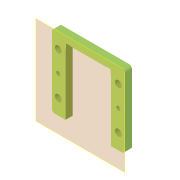
# Autodesk Inventor part: 30_Linear_Stage_NEMA11_China_lid_universal_extender_v2
Saved by Autodesk Inventor 2022 (Build 260153000, 153)
## iProperties
Created: 2022-02-11
Part Number: 30_Linear_Stage_NEMA11_China_lid_universal_extender_v2
Material: Generic
Document SubType Name: Modeling
Designer: wanghaoran
Density: 1 g/cm^3
Appearance: ipht green
Catalog Web Link: isPrinted
Vendor: openUC2
Mass: 6.04917 g
Surface Area: 45.2263 cm^2
Volume: 6.04917 cm^3
Author: wanghaoran
Autodesk Inventor part; units mm, degrees
ref_plane "YZ Plane" through (0, 0, 0) normal (1, 0, 0) x (0, 1, 0)
ref_plane "XZ Plane" through (0, 0, 0) normal (0, 1, 0) x (-1, 0, 0)
ref_plane "XY Plane" through (0, 0, 0) normal (0, 0, 1) x (1, 0, 0)
sketch "Sketch1" plane through (0, 0, 0) normal (0, 0, 1) x (1, 0, 0)
  circle A0 centre (-21, 1.215) radius 1.4 projected
  circle A1 centre (21, 1.215) radius 1.4 projected
  arc A2 (24.9, 3.115) -> (22.9, 5.115) centre (22.9, 3.115) ccw projected
  line L0 (22.9, 5.115) -> (-22.9, 5.115) projected
  arc A3 (-22.9, 5.115) -> (-24.9, 3.115) centre (-22.9, 3.115) ccw projected
  line L1 (-24.9, 3.115) -> (-24.9, -5.115) projected
  line L2 (22.8395, -5.115) -> (24.9, -5.115) projected
  line L3 (24.9, -5.115) -> (24.9, 3.115) projected
  arc A4 (22.9, -44.685) -> (24.9, -42.685) centre (22.9, -42.685) ccw projected
  line L4 (24.9, -42.685) -> (24.9, -36.885) projected
  line L5 (24.9, -36.885) -> (17.1, -36.885) projected
  line L6 (17.1, -36.885) -> (17.1, -44.685) projected
  line L7 (17.1, -44.685) -> (22.9, -44.685) projected
  circle A5 centre (21, -40.785) radius 1.4 projected
  arc A6 (-24.9, -42.685) -> (-22.9, -44.685) centre (-22.9, -42.685) ccw projected
  line L8 (-22.9, -44.685) -> (-17.1, -44.685) projected
  line L9 (-17.1, -44.685) -> (-17.1, -36.885) projected
  line L10 (-17.1, -36.885) -> (-24.9, -36.885) projected
  line L11 (-24.9, -36.885) -> (-24.9, -42.685) projected
  circle A7 centre (-21, -40.785) radius 1.4 projected
  line L12 (24.9, 5.115) -> (-24.9, 5.115)
  line L13 (-24.9, 5.115) -> (-24.9, -44.685)
  line L14 (-24.9, -44.685) -> (24.9, -44.685)
  line L15 (24.9, -44.685) -> (24.9, 5.115)
  line L16 (17.1, -2.685) -> (-17.1, -2.685)
  line L17 (-17.1, -2.685) -> (-17.1, -36.885)
  line L18 (-17.1, -36.885) -> (17.1, -36.885)
  line L19 (17.1, -36.885) -> (17.1, -2.685)
  line L20 (17.1, -36.885) -> (17.1, -44.685)
  line L21 (-17.1, -36.885) -> (-17.1, -44.685)
  circle A8 centre (0, 1.415) radius 1.4 projected
  arc A9 (-18.2605, -5.115) -> (-22.8395, -5.115) centre (-20.55, -5.335) ccw projected
  arc A10 (22.8395, -5.115) -> (18.2605, -5.115) centre (20.55, -5.335) ccw projected
  circle A11 centre (14.45, 0.765) radius 2.3 projected
  circle A12 centre (-14.45, 0.765) radius 2.3 projected
  line L22 (-24.9, -5.115) -> (-22.8395, -5.115) projected
  line L23 (-18.2605, -5.115) -> (18.2605, -5.115) projected
  circle A13 centre (20, -39.785) radius 1.4 projected
  circle A14 centre (-20, -39.785) radius 1.4 projected
  circle A15 centre (-14.45, -40.335) radius 2.3 projected
  circle A16 centre (20.55, -34.235) radius 2.3 projected
  circle A17 centre (-20.55, -34.235) radius 2.3 projected
  circle A18 centre (14.45, -40.335) radius 2.3 projected
  arc A19 (22.9, -44.685) -> (24.9, -42.685) centre (22.9, -42.685) ccw projected
  line L24 (24.9, -42.685) -> (24.9, -4.885) projected
  line L25 (24.9, -4.885) -> (22.8055, -4.885) projected
  line L26 (17.1, -4.885) -> (17.1, -36.885) projected
  line L27 (17.1, -36.885) -> (-17.1, -36.885) projected
  line L28 (-17.1, -36.885) -> (-17.1, -4.885) projected
  line L29 (-22.8055, -4.885) -> (-24.9, -4.885) projected
  line L30 (-24.9, -4.885) -> (-24.9, -42.685) projected
  arc A20 (-24.9, -42.685) -> (-22.9, -44.685) centre (-22.9, -42.685) ccw projected
  line L31 (-22.9, -44.685) -> (22.9, -44.685) projected
  arc A21 (-22.8055, -4.885) -> (-18.2945, -4.885) centre (-20.55, -5.335) ccw projected
  arc A22 (18.2945, -4.885) -> (22.8055, -4.885) centre (20.55, -5.335) ccw projected
  line L32 (18.2945, -4.885) -> (17.1, -4.885) projected
  line L33 (-17.1, -4.885) -> (-18.2945, -4.885) projected
  line L34 (17.1, -44.685) -> (15.6, -44.685)
  line L35 (15.6, -44.685) -> (15.6, -2.685)
  line L36 (15.6, -2.685) -> (17.1, -2.685)
  line L37 (17.1, -2.685) -> (17.1, -44.685)
  line L38 (-17.1, -44.685) -> (-15.6, -44.685)
  line L39 (-15.6, -44.685) -> (-15.6, -2.685)
  line L40 (-15.6, -2.685) -> (-17.1, -2.685)
  line L41 (-17.1, -2.685) -> (-17.1, -44.685)
  line L42 (-15, -27.435) -> (15, -27.435) projected
  line L43 (15, -27.435) -> (15, 0.565) projected
  line L44 (15, 0.565) -> (-15, 0.565) projected
  line L45 (-15, 0.565) -> (-15, -27.435) projected
  circle A23 centre (0, -19.785) radius 6.5 projected
  circle A24 centre (-10, -2.435) radius 2.75 projected
  circle A25 centre (10, -2.435) radius 2.75 projected
  line L46 (15.2, 0.765) -> (15.2, -27.635)
  line L47 (15.2, -27.635) -> (-15.2, -27.635)
  line L48 (-15.2, -27.635) -> (-15.2, 0.765)
  line L49 (-15.2, 0.765) -> (15.2, 0.765)
  point P0 (0, 0)
  point P1 (-20.55, -5.335)
  point P2 (20.55, -5.335)
  point P3 (-20.55, -5.335)
  point P4 (20.55, -5.335)
  point P5 (15.2, -2.685)
  point P6 (-15.2, -2.685)
  point P7 (-12.15, 0.765)
  point P8 (-12.1587, 0.565)
  point P9 (12.1587, 0.565)
  point P10 (12.15, 0.765)
  point P11 (-15.6, -36.885)
  point P12 (15.6, -36.885)
  dimension "d0" = 7.8
  dimension "d23" = 1.5
  dimension "d24" = 1.5
  dimension "d57" = 0.2
  constraints: 44 end point, 10 equal length, 7 point on line, 4 perpendicular, 3 horizontal, 6 other
  measures "d0" distance between parallel lines of L15 L19
  measures "d23" distance between parallel lines of L6 L35
  measures "d24" distance between parallel lines of L39 L28
  measures "d57" distance between parallel lines of L43 L46
extrude "Extrusion1" add sketch "Sketch1" along normal blind 5 contours A0 | A1 | L3 L25 A10 L32 L19 L16 L46 A11 L49 A8 A12 L48 L17 L33 A9 L29 L1 A3 L0 A2 | L3 L2 A10 L25 | L15 L5 L19 L23 A22 L2 | A10 A22 | L4 A4 L7 L6 L5 | A10 L23 L19 L32 | L29 A9 L22 L1 | L6 L14 L35 A18 L18 | L18 L35 L23 L19 | L19 L23 L35 L16 | L22 A21 L23 L17 L10 L13 | A9 A21 | L10 L9 L8 A6 L11 | L33 L17 L23 A9 | L39 A15 L14 L9 L18 | L18 L17 L23 L39 | A18 L35 | L17 L16 L39 L23 | L39 A15 | L46 L49 A11 | A12 L49 L48 | L44 A8 L49 A11 | L49 A8 L44 A12 | L44 A8 L49 | L49 A8 | A5 A13 | A13 A5 | A5 A13 | A7 A14 | A7 A14 | A14 A7 | A16 | A17 picked at (16.0467, -40.1174) picked at (-15.7428, -39.7773)
ref_plane "Arbeitsebene1" through (15.3065, -4.4785, 13.1) normal (0, 0, 1) x (0, 1, 0)
sketch "Skizze3" plane through (15.3065, -4.4785, 13.1) normal (0, 0, 1) x (0, 1, 0)
  line L0 (-0.0065, 32.6065) -> (-30.6065, 32.6065) projected
  arc A0 (1.9935, 30.6065) -> (-0.0065, 32.6065) centre (-0.0065, 30.6065) ccw projected
  line L1 (1.9935, 30.6065) -> (1.9935, 0.0065) projected
  arc A1 (-0.0065, -1.9935) -> (1.9935, 0.0065) centre (-0.0065, 0.0065) ccw projected
  line L2 (-0.0065, -1.9935) -> (-30.6065, -1.9935) projected
  arc A2 (-32.6065, 0.0065) -> (-30.6065, -1.9935) centre (-30.6065, 0.0065) ccw projected
  line L3 (-32.6065, 0.0065) -> (-32.6065, 30.6065) projected
  arc A3 (-30.6065, 32.6065) -> (-32.6065, 30.6065) centre (-30.6065, 30.6065) ccw projected
  circle A4 centre (-35.2065, 35.2065) radius 2.4 projected
  circle A5 centre (-35.8565, 29.7565) radius 2.45 projected
  circle A6 centre (-29.7565, 35.8565) radius 2.45 projected
  circle A7 centre (-35.2065, -4.5935) radius 2.4 projected
  circle A8 centre (-35.8565, 0.8565) radius 2.45 projected
  circle A9 centre (-29.7565, -5.2435) radius 2.45 projected
  circle A10 centre (4.5935, 35.2065) radius 2.4 projected
  circle A11 centre (5.2435, 29.7565) radius 2.45 projected
  circle A12 centre (-0.8565, 35.8565) radius 2.45 projected
  circle A13 centre (-0.8565, -5.2435) radius 2.45 projected
  circle A14 centre (5.2435, 0.8565) radius 2.45 projected
  circle A15 centre (4.5935, -4.5935) radius 2.4 projected
  line L4 (-10.3065, -9.6935) -> (7.6935, -9.6935) projected
  arc A16 (7.6935, -9.6935) -> (9.6935, -7.6935) centre (7.6935, -7.6935) ccw projected
  line L5 (9.6935, 10.3065) -> (9.6935, -7.6935) projected
  line L6 (9.6935, 10.3065) -> (10.5197, 10.3065) projected
  arc A17 (10.9935, 9.9665) -> (10.5197, 10.3065) centre (10.5197, 9.8065) ccw projected
  arc A18 (10.9935, 9.9665) -> (12.953, 8.3665) centre (12.953, 10.3665) ccw projected
  line L7 (12.953, 8.3665) -> (13.0935, 8.3665) projected
  arc A19 (13.0935, 8.3665) -> (15.0935, 10.3665) centre (13.0935, 10.3665) ccw projected
  line L8 (15.0935, 10.3665) -> (15.0935, 20.2465) projected
  arc A20 (15.0935, 20.2465) -> (13.0935, 22.2465) centre (13.0935, 20.2465) ccw projected
  line L9 (13.0935, 22.2465) -> (12.953, 22.2465) projected
  arc A21 (12.953, 22.2465) -> (10.9935, 20.6465) centre (12.953, 20.2465) ccw projected
  arc A22 (10.5197, 20.3065) -> (10.9935, 20.6465) centre (10.5197, 20.8065) ccw projected
  line L10 (10.5197, 20.3065) -> (9.6935, 20.3065) projected
  line L11 (9.6935, 38.3065) -> (9.6935, 20.3065) projected
  arc A23 (9.6935, 38.3065) -> (7.6935, 40.3065) centre (7.6935, 38.3065) ccw projected
  line L12 (7.6935, 40.3065) -> (-10.156, 40.3065) projected
  line L13 (-10.156, 40.3065) -> (-10.1563, 39.5805) projected
  arc A24 (-10.1563, 39.5805) -> (-9.9265, 39.2516) centre (-9.8062, 39.5805) ccw projected
  arc A25 (-8.2165, 37.1473) -> (-9.9265, 39.2516) centre (-10.3665, 37.1472) ccw projected
  line L14 (-8.2165, 37.1473) -> (-8.2165, 37.007) projected
  arc A26 (-10.3664, 34.8569) -> (-8.2165, 37.007) centre (-10.3665, 37.0069) ccw projected
  line L15 (-10.3664, 34.8569) -> (-20.25, 34.8563) projected
  arc A27 (-22.4012, 37.0074) -> (-20.25, 34.8563) centre (-20.2501, 37.0074) ccw projected
  line L16 (-22.4012, 37.0074) -> (-22.4012, 37.1472) projected
  arc A28 (-20.6871, 39.2564) -> (-22.4012, 37.1472) centre (-20.2465, 37.1472) ccw projected
  arc A29 (-20.6871, 39.2564) -> (-20.4574, 39.5808) centre (-20.8064, 39.5844) ccw projected
  line L17 (-20.4574, 39.5808) -> (-20.4576, 40.3065) projected
  line L18 (-20.4576, 40.3065) -> (-38.3065, 40.3065) projected
  arc A30 (-38.3065, 40.3065) -> (-40.3065, 38.3065) centre (-38.3065, 38.3065) ccw projected
  line L19 (-40.3065, 20.4571) -> (-40.3065, 38.3065) projected
  line L20 (-40.3065, 20.4571) -> (-39.5805, 20.4567) projected
  arc A31 (-39.5805, 20.4567) -> (-39.2516, 20.6865) centre (-39.5805, 20.8069) ccw projected
  arc A32 (-37.1473, 22.3966) -> (-39.2516, 20.6865) centre (-37.1472, 20.2466) ccw projected
  line L21 (-37.1473, 22.3966) -> (-37.007, 22.3966) projected
  arc A33 (-34.8569, 20.2467) -> (-37.007, 22.3966) centre (-37.0069, 20.2466) ccw projected
  line L22 (-34.8569, 20.2467) -> (-34.8563, 10.3631) projected
  arc A34 (-37.0074, 8.2119) -> (-34.8563, 10.3631) centre (-37.0074, 10.363) ccw projected
  line L23 (-37.0074, 8.2119) -> (-37.1472, 8.2119) projected
  arc A35 (-39.2564, 9.9259) -> (-37.1472, 8.2119) centre (-37.1472, 10.3665) ccw projected
  arc A36 (-39.2564, 9.9259) -> (-39.5808, 10.1556) centre (-39.5844, 9.8067) ccw projected
  line L24 (-39.5808, 10.1556) -> (-40.3065, 10.1554) projected
  line L25 (-40.3065, -7.6935) -> (-40.3065, 10.1554) projected
  arc A37 (-40.3065, -7.6935) -> (-38.3065, -9.6935) centre (-38.3065, -7.6935) ccw projected
  line L26 (-38.3065, -9.6935) -> (-20.3065, -9.6935) projected
  line L27 (-20.3065, -9.6935) -> (-20.3065, -10.5197) projected
  arc A38 (-20.6465, -10.9935) -> (-20.3065, -10.5197) centre (-20.8065, -10.5197) ccw projected
  arc A39 (-20.6465, -10.9935) -> (-22.2465, -12.953) centre (-20.2465, -12.953) ccw projected
  line L28 (-22.2465, -12.953) -> (-22.2465, -13.0935) projected
  arc A40 (-22.2465, -13.0935) -> (-20.2465, -15.0935) centre (-20.2465, -13.0935) ccw projected
  line L29 (-20.2465, -15.0935) -> (-10.3665, -15.0935) projected
  arc A41 (-10.3665, -15.0935) -> (-8.3665, -13.0935) centre (-10.3665, -13.0935) ccw projected
  line L30 (-8.3665, -13.0935) -> (-8.3665, -12.953) projected
  arc A42 (-8.3665, -12.953) -> (-9.9665, -10.9935) centre (-10.3665, -12.953) ccw projected
  arc A43 (-10.3065, -10.5197) -> (-9.9665, -10.9935) centre (-9.8065, -10.5197) ccw projected
  line L31 (-10.3065, -10.5197) -> (-10.3065, -9.6935) projected
  circle A44 centre (-15.4065, -5.9935) radius 2.15 projected
  circle A45 centre (5.9935, 15.2065) radius 2.15 projected
  point P0 (4.4785, 15.3065)
hole "Bohrung1" at (-20.55, -34.235, 13.1) at (-20.55, -5.335, 13.1) at (20.55, -5.335, 13.1) at (20.55, -34.235, 13.1) direction (0, 0, -1) diameter 4.6 end through all
sketch "Skizze10" plane through (0, 0, 0) normal (0, 0, -1) x (-1, 0, 0)
  circle A0 centre (-20.55, -19.785) radius 1.4 projected
  circle A1 centre (20.55, -19.785) radius 1.4 projected
  point P0 (0, 0)
hole "Bohrung5" at (20.55, -19.785, 0) at (-20.55, -19.785, 0) direction (0, 0, 1) diameter 2.8 end through all counterbore diameter 6 counterbore depth 3
body "Solid1"
